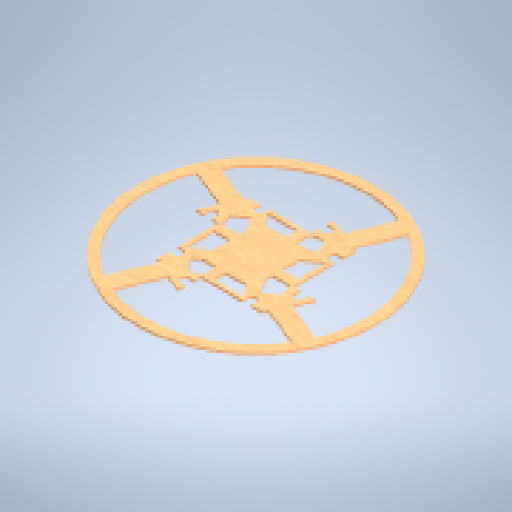
# Autodesk Inventor part: plate
Saved by Autodesk Inventor 2024.1 (Build 281209000, 209)
## iProperties
Created: 2024-07-03
Part Number: plate
Material: 木材 (サクラ材)
Document SubType Name: Modeling
Designer: hibik
Density: 0.63 g/cm^3
Appearance: サクラ材 - ナチュラル 抑えた光沢
Author: hibik
Autodesk Inventor part; units mm, degrees
ref_plane "YZ Plane" through (0, 0, 0) normal (1, 0, 0) x (0, 1, 0)
ref_plane "XZ Plane" through (0, 0, 0) normal (0, 1, 0) x (-1, 0, 0)
ref_plane "XY Plane" through (0, 0, 0) normal (0, 0, 1) x (1, 0, 0)
sketch "スケッチ1" plane through (0, 0, 0) normal (0, 1, 0) x (-1, 0, 0)
  line L0 (26.5, 31.5) -> (-26.5, 31.5)
  line L1 (-26.5, 31.5) -> (-26.5, -31.5)
  line L2 (-26.5, -31.5) -> (26.5, -31.5)
  line L3 (26.5, -31.5) -> (26.5, 31.5)
  line L4 (26.5, 31.5) -> (-26.5, -31.5) construction
  line L5 (-26.5, 31.5) -> (26.5, -31.5) construction
  point P0 (0, 0)
  dimension "d0" = 53
  dimension "d1" = 63
  constraints: 12 end point, 2 midpoint, 2 parallel, 1 horizontal, 1 perpendicular
  measures "d0" distance of L2.end L1.end
  measures "d1" distance of L1.end L0.end
extrude "押し出し1" add sketch "スケッチ1" along normal blind 2.5
sketch "スケッチ6" plane through (0, 0, 0) normal (0, -1, 0) x (1, 0, 0)
  arc A0 (26.3287, -65.2977) -> (29.0118, -58.5429) centre (24.4787, -60.6525) ccw projected
  line L0 (26.3287, -65.2977) -> (44.15, -58.2) projected
  line L1 (44.15, -54.8) -> (44.15, -58.2) projected
  line L2 (46.15, -54.8) -> (44.15, -54.8) projected
  line L3 (46.15, -54.8) -> (48, -54.8) projected
  line L4 (48, -43.3721) -> (48, -54.8) projected
  line L5 (48, -43.3721) -> (43, -43.3721) projected
  arc A1 (40.1241, -42.4623) -> (43, -43.3721) centre (43, -38.3721) ccw projected
  line L6 (40.1241, -42.4623) -> (42.3111, -44) projected
  arc A2 (36.5717, -56.5915) -> (42.3111, -44) centre (32.8717, -47.3012) ccw projected
  line L7 (36.5717, -56.5915) -> (32.1435, -58.3551) projected
  arc A3 (29.0118, -58.5429) -> (32.1435, -58.3551) centre (30.2935, -53.7099) ccw projected
  line L8 (-26.5, 18.6328) -> (-26.5, 0) projected
  line L9 (-26.5, 0) -> (-44, 0) projected
  line L10 (-44, 0) -> (-44, 30.9375) projected
  line L11 (-44, 30.9375) -> (-26.5, 18.6328) projected
  line L12 (22.5, 27.5) -> (22.5, -27.5) projected
  line L13 (22.5, -27.5) -> (-22.5, -27.5) projected
  line L14 (-22.5, -27.5) -> (-22.5, 27.5) projected
  line L15 (-22.5, 27.5) -> (22.5, 27.5) projected
  line L16 (22.1484, 31.5) -> (0, 31.5) projected
  line L17 (0, 31.5) -> (0, 44) projected
  line L18 (0, 44) -> (30.9375, 44) projected
  line L19 (30.9375, 44) -> (22.1484, 31.5) projected
  line L20 (26.5, -18.6328) -> (26.5, 0) projected
  line L21 (26.5, 0) -> (44, 0) projected
  line L22 (44, 0) -> (44, -30.9375) projected
  line L23 (44, -30.9375) -> (26.5, -18.6328) projected
  line L24 (-22.1484, -31.5) -> (0, -31.5) projected
  line L25 (0, -31.5) -> (0, -44) projected
  line L26 (0, -44) -> (-30.9375, -44) projected
  line L27 (-30.9375, -44) -> (-22.1484, -31.5) projected
  arc A4 (25.7604, -55.8196) -> (19.4893, -60.3263) centre (24.4787, -60.6525) ccw projected
  arc A5 (25.6484, -55.56) -> (25.7604, -55.8196) centre (30.2935, -53.7099) ccw projected
  arc A6 (25.6484, -55.56) -> (14.5, -48) centre (14.5, -60) ccw projected
  arc A7 (9.5, -43) -> (14.5, -48) centre (14.5, -43) ccw projected
  line L28 (9.5, -43) -> (9.5, -31.5) projected
  line L29 (9.5, -31.5) -> (24.5333, -31.5) projected
  line L30 (24.5333, -31.5) -> (40.1241, -42.4623) projected
  arc A8 (39.1622, -35.1673) -> (40.1241, -42.4623) centre (43, -38.3721) ccw projected
  circle A9 centre (35.3243, -31.9624) radius 5 projected
  arc A10 (43, -33.3721) -> (39.1622, -35.1673) centre (43, -38.3721) ccw projected
  line L31 (43, -33.3721) -> (48, -33.3721) projected
  line L32 (48, -19.5) -> (48, -33.3721) projected
  line L33 (50, -19.5) -> (48, -19.5) projected
  line L34 (50, -19.5) -> (50, 4.5) projected
  line L35 (48, 4.5) -> (50, 4.5) projected
  line L36 (48, 9.5) -> (48, 4.5) projected
  line L37 (53, 9.5) -> (48, 9.5) projected
  line L38 (53, 7.5) -> (53, 9.5) projected
  line L39 (53, 7.5) -> (67, 7.5) projected
  line L40 (67, 9.5) -> (67, 7.5) projected
  line L41 (72, 9.5) -> (67, 9.5) projected
  line L42 (72, 9.5) -> (65.2977, 26.3287) projected
  arc A11 (60.3263, 19.4893) -> (65.2977, 26.3287) centre (60.6525, 24.4787) ccw projected
  circle A12 centre (60, 14.5) radius 5 projected
  arc A13 (55.8196, 25.7604) -> (60.3263, 19.4893) centre (60.6525, 24.4787) ccw projected
  arc A14 (55.56, 25.6484) -> (55.8196, 25.7604) centre (53.7099, 30.2935) ccw projected
  arc A15 (55.56, 25.6484) -> (48, 14.5) centre (60, 14.5) ccw projected
  arc A16 (43, 9.5) -> (48, 14.5) centre (43, 14.5) ccw projected
  line L43 (43, 9.5) -> (26.5, 9.5) projected
  line L44 (26.5, 9.5) -> (26.5, 17.4222) projected
  line L45 (26.5, 17.4222) -> (42.4623, 40.1241) projected
  arc A17 (35.1673, 39.1622) -> (42.4623, 40.1241) centre (38.3721, 43) ccw projected
  circle A18 centre (31.9624, 35.3243) radius 5 projected
  arc A19 (33.3721, 43) -> (35.1673, 39.1622) centre (38.3721, 43) ccw projected
  line L46 (33.3721, 43) -> (33.3721, 48) projected
  line L47 (19.5, 48) -> (33.3721, 48) projected
  line L48 (19.5, 50) -> (19.5, 48) projected
  line L49 (19.5, 50) -> (-4.5, 50) projected
  line L50 (-4.5, 48) -> (-4.5, 50) projected
  line L51 (-9.5, 48) -> (-4.5, 48) projected
  line L52 (-9.5, 53) -> (-9.5, 48) projected
  line L53 (-7.5, 53) -> (-9.5, 53) projected
  line L54 (-7.5, 53) -> (-7.5, 67) projected
  line L55 (-9.5, 67) -> (-7.5, 67) projected
  line L56 (-9.5, 72) -> (-9.5, 67) projected
  line L57 (-9.5, 72) -> (-26.3287, 65.2977) projected
  arc A20 (-19.4893, 60.3263) -> (-26.3287, 65.2977) centre (-24.4787, 60.6525) ccw projected
  circle A21 centre (-14.5, 60) radius 5 projected
  arc A22 (-25.7604, 55.8196) -> (-19.4893, 60.3263) centre (-24.4787, 60.6525) ccw projected
  arc A23 (-25.6484, 55.56) -> (-25.7604, 55.8196) centre (-30.2935, 53.7099) ccw projected
  arc A24 (-25.6484, 55.56) -> (-14.5, 48) centre (-14.5, 60) ccw projected
  arc A25 (-9.5, 43) -> (-14.5, 48) centre (-14.5, 43) ccw projected
  line L58 (-9.5, 43) -> (-9.5, 31.5) projected
  line L59 (-9.5, 31.5) -> (-24.5333, 31.5) projected
  line L60 (-24.5333, 31.5) -> (-40.1241, 42.4623) projected
  arc A26 (-39.1622, 35.1673) -> (-40.1241, 42.4623) centre (-43, 38.3721) ccw projected
  circle A27 centre (-35.3243, 31.9624) radius 5 projected
  arc A28 (-43, 33.3721) -> (-39.1622, 35.1673) centre (-43, 38.3721) ccw projected
  line L61 (-43, 33.3721) -> (-48, 33.3721) projected
  line L62 (-48, 19.5) -> (-48, 33.3721) projected
  line L63 (-50, 19.5) -> (-48, 19.5) projected
  line L64 (-50, 19.5) -> (-50, -4.5) projected
  line L65 (-48, -4.5) -> (-50, -4.5) projected
  line L66 (-48, -9.5) -> (-48, -4.5) projected
  line L67 (-53, -9.5) -> (-48, -9.5) projected
  line L68 (-53, -7.5) -> (-53, -9.5) projected
  line L69 (-53, -7.5) -> (-67, -7.5) projected
  line L70 (-67, -9.5) -> (-67, -7.5) projected
  line L71 (-72, -9.5) -> (-67, -9.5) projected
  line L72 (-72, -9.5) -> (-65.2977, -26.3287) projected
  arc A29 (-60.3263, -19.4893) -> (-65.2977, -26.3287) centre (-60.6525, -24.4787) ccw projected
  circle A30 centre (-60, -14.5) radius 5 projected
  arc A31 (-55.8196, -25.7604) -> (-60.3263, -19.4893) centre (-60.6525, -24.4787) ccw projected
  arc A32 (-55.56, -25.6484) -> (-55.8196, -25.7604) centre (-53.7099, -30.2935) ccw projected
  arc A33 (-55.56, -25.6484) -> (-48, -14.5) centre (-60, -14.5) ccw projected
  arc A34 (-43, -9.5) -> (-48, -14.5) centre (-43, -14.5) ccw projected
  line L73 (-43, -9.5) -> (-26.5, -9.5) projected
  line L74 (-26.5, -9.5) -> (-26.5, -17.4222) projected
  line L75 (-26.5, -17.4222) -> (-42.4623, -40.1241) projected
  arc A35 (-35.1673, -39.1622) -> (-42.4623, -40.1241) centre (-38.3721, -43) ccw projected
  circle A36 centre (-31.9624, -35.3243) radius 5 projected
  arc A37 (-33.3721, -43) -> (-35.1673, -39.1622) centre (-38.3721, -43) ccw projected
  line L76 (-33.3721, -43) -> (-33.3721, -48) projected
  line L77 (-19.5, -48) -> (-33.3721, -48) projected
  line L78 (-19.5, -50) -> (-19.5, -48) projected
  line L79 (-19.5, -50) -> (4.5, -50) projected
  line L80 (4.5, -48) -> (4.5, -50) projected
  line L81 (9.5, -48) -> (4.5, -48) projected
  line L82 (9.5, -53) -> (9.5, -48) projected
  line L83 (7.5, -53) -> (9.5, -53) projected
  line L84 (7.5, -53) -> (7.5, -67) projected
  line L85 (9.5, -67) -> (7.5, -67) projected
  line L86 (9.5, -72) -> (9.5, -67) projected
  line L87 (9.5, -72) -> (26.3287, -65.2977) projected
  arc A38 (19.4893, -60.3263) -> (26.3287, -65.2977) centre (24.4787, -60.6525) ccw projected
  circle A39 centre (14.5, -60) radius 5 projected
  arc A40 (-65.2977, -26.3287) -> (-58.5429, -29.0118) centre (-60.6525, -24.4787) ccw projected
  line L88 (-65.2977, -26.3287) -> (-58.2, -44.15) projected
  line L89 (-54.8, -44.15) -> (-58.2, -44.15) projected
  line L90 (-54.8, -46.15) -> (-54.8, -44.15) projected
  line L91 (-54.8, -46.15) -> (-54.8, -48) projected
  line L92 (-43.3721, -48) -> (-54.8, -48) projected
  line L93 (-43.3721, -48) -> (-43.3721, -43) projected
  arc A41 (-42.4623, -40.1241) -> (-43.3721, -43) centre (-38.3721, -43) ccw projected
  line L94 (-42.4623, -40.1241) -> (-44, -42.3111) projected
  arc A42 (-56.5915, -36.5717) -> (-44, -42.3111) centre (-47.3012, -32.8717) ccw projected
  line L95 (-56.5915, -36.5717) -> (-58.3551, -32.1435) projected
  arc A43 (-58.5429, -29.0118) -> (-58.3551, -32.1435) centre (-53.7099, -30.2935) ccw projected
  arc A44 (-26.3287, 65.2977) -> (-29.0118, 58.5429) centre (-24.4787, 60.6525) ccw projected
  line L96 (-26.3287, 65.2977) -> (-44.15, 58.2) projected
  line L97 (-44.15, 54.8) -> (-44.15, 58.2) projected
  line L98 (-46.15, 54.8) -> (-44.15, 54.8) projected
  line L99 (-46.15, 54.8) -> (-48, 54.8) projected
  line L100 (-48, 43.3721) -> (-48, 54.8) projected
  line L101 (-48, 43.3721) -> (-43, 43.3721) projected
  arc A45 (-40.1241, 42.4623) -> (-43, 43.3721) centre (-43, 38.3721) ccw projected
  line L102 (-40.1241, 42.4623) -> (-42.3111, 44) projected
  arc A46 (-36.5717, 56.5915) -> (-42.3111, 44) centre (-32.8717, 47.3012) ccw projected
  line L103 (-36.5717, 56.5915) -> (-32.1435, 58.3551) projected
  arc A47 (-29.0118, 58.5429) -> (-32.1435, 58.3551) centre (-30.2935, 53.7099) ccw projected
  arc A48 (65.2977, 26.3287) -> (58.5429, 29.0118) centre (60.6525, 24.4787) ccw projected
  line L104 (65.2977, 26.3287) -> (58.2, 44.15) projected
  line L105 (54.8, 44.15) -> (58.2, 44.15) projected
  line L106 (54.8, 46.15) -> (54.8, 44.15) projected
  line L107 (54.8, 46.15) -> (54.8, 48) projected
  line L108 (43.3721, 48) -> (54.8, 48) projected
  line L109 (43.3721, 48) -> (43.3721, 43) projected
  arc A49 (42.4623, 40.1241) -> (43.3721, 43) centre (38.3721, 43) ccw projected
  line L110 (42.4623, 40.1241) -> (44, 42.3111) projected
  arc A50 (56.5915, 36.5717) -> (44, 42.3111) centre (47.3012, 32.8717) ccw projected
  line L111 (56.5915, 36.5717) -> (58.3551, 32.1435) projected
  arc A51 (58.5429, 29.0118) -> (58.3551, 32.1435) centre (53.7099, 30.2935) ccw projected
  line L112 (35.3243, -31.9624) -> (14.5, -60)
  line L113 (-31.9624, -35.3243) -> (-60, -14.5)
  line L114 (-35.3243, 31.9624) -> (-14.5, 60)
  line L115 (60, 14.5) -> (31.9624, 35.3243)
  line L116 (-48, -9.5) -> (-48, 33.3721) projected
  line L117 (9.5, -48) -> (-33.3721, -48) projected
  line L118 (48, 9.5) -> (48, -33.3721) projected
  line L119 (-9.5, 48) -> (33.3721, 48) projected
  circle A52 centre (-60, -14.5) radius 1.55 projected
  circle A53 centre (-43, 38.3721) radius 1.55 projected
  circle A54 centre (-71.5, 53.2) radius 1.55 projected
  line L120 (-51.7493, 27.3) -> (-63.2507, 27.3) projected
  line L121 (-63.2507, 27.3) -> (-57.5, 36.8845) projected
  line L122 (-57.5, 36.8845) -> (-51.7493, 27.3) projected
  line L123 (-50, -4.5) -> (-57.5556, 7.5) projected
  line L124 (-57.5556, 7.5) -> (-50, 19.5) projected
  line L125 (-50, 19.5) -> (-50, -4.5) projected
  line L126 (-70, 19.5) -> (-62.4444, 7.5) projected
  line L127 (-62.4444, 7.5) -> (-70, -4.5) projected
  line L128 (-70, -4.5) -> (-70, 19.5) projected
  line L129 (-50, 49.3845) -> (-50, 30.2155) projected
  line L130 (-50, 30.2155) -> (-55.7507, 39.8) projected
  line L131 (-55.7507, 39.8) -> (-50, 49.3845) projected
  line L132 (-59.2493, 39.8) -> (-65, 30.2155) projected
  line L133 (-65, 30.2155) -> (-65, 49.3845) projected
  line L134 (-65, 49.3845) -> (-59.2493, 39.8) projected
  line L135 (-53, 22.5) -> (-60, 11.3824) projected
  line L136 (-60, 11.3824) -> (-67, 22.5) projected
  line L137 (-67, 22.5) -> (-53, 22.5) projected
  line L138 (-67, -7.5) -> (-60, 3.6176) projected
  line L139 (-60, 3.6176) -> (-53, -7.5) projected
  line L140 (-53, -7.5) -> (-67, -7.5) projected
  line L141 (-51.7493, 52.3) -> (-57.5, 42.7155) projected
  line L142 (-57.5, 42.7155) -> (-63.2507, 52.3) projected
  line L143 (-63.2507, 52.3) -> (-51.7493, 52.3) projected
  line L144 (-66.5, 58.3) -> (-66.5, 58.2) projected
  line L145 (-66.5, 58.2) -> (-71.5, 58.2) projected
  arc A55 (-71.5, 58.2) -> (-71.5, 48.2) centre (-71.5, 53.2) ccw projected
  line L146 (-71.5, 48.2) -> (-66.5, 48.2) projected
  line L147 (-66.5, 48.2) -> (-66.5, 27.3) projected
  line L148 (-66.5, 27.3) -> (-72, 27.3) projected
  line L149 (-72, 27.3) -> (-72, -9.5) projected
  line L150 (-72, -9.5) -> (-65, -9.5) projected
  line L151 (-65, -9.5) -> (-65, -14.5) projected
  arc A56 (-65, -14.5) -> (-55, -14.5) centre (-60, -14.5) ccw projected
  line L152 (-55, -14.5) -> (-55, -9.5) projected
  line L153 (-55, -9.5) -> (-48, -9.5) projected
  line L154 (-48, -9.5) -> (-48, 33.3721) projected
  line L155 (-48, 33.3721) -> (-43, 33.3721) projected
  arc A57 (-43, 33.3721) -> (-43, 43.3721) centre (-43, 38.3721) ccw projected
  line L156 (-43, 43.3721) -> (-48, 43.3721) projected
  line L157 (-48, 43.3721) -> (-48, 54.8) projected
  line L158 (-48, 54.8) -> (-44.1513, 54.8) projected
  line L159 (-44.1513, 58.3) -> (-44.1513, 54.8) projected
  line L160 (-66.5, 58.3) -> (-44.1513, 58.3) projected
  circle A58 centre (14.5, -60) radius 1.55 projected
  circle A59 centre (-38.3721, -43) radius 1.55 projected
  circle A60 centre (-53.2, -71.5) radius 1.55 projected
  line L161 (-27.3, -51.7493) -> (-27.3, -63.2507) projected
  line L162 (-27.3, -63.2507) -> (-36.8845, -57.5) projected
  line L163 (-36.8845, -57.5) -> (-27.3, -51.7493) projected
  line L164 (4.5, -50) -> (-7.5, -57.5556) projected
  line L165 (-7.5, -57.5556) -> (-19.5, -50) projected
  line L166 (-19.5, -50) -> (4.5, -50) projected
  line L167 (-19.5, -70) -> (-7.5, -62.4444) projected
  line L168 (-7.5, -62.4444) -> (4.5, -70) projected
  line L169 (4.5, -70) -> (-19.5, -70) projected
  line L170 (-49.3845, -50) -> (-30.2155, -50) projected
  line L171 (-30.2155, -50) -> (-39.8, -55.7507) projected
  line L172 (-39.8, -55.7507) -> (-49.3845, -50) projected
  line L173 (-39.8, -59.2493) -> (-30.2155, -65) projected
  line L174 (-30.2155, -65) -> (-49.3845, -65) projected
  line L175 (-49.3845, -65) -> (-39.8, -59.2493) projected
  line L176 (-22.5, -53) -> (-11.3824, -60) projected
  line L177 (-11.3824, -60) -> (-22.5, -67) projected
  line L178 (-22.5, -67) -> (-22.5, -53) projected
  line L179 (7.5, -67) -> (-3.6176, -60) projected
  line L180 (-3.6176, -60) -> (7.5, -53) projected
  line L181 (7.5, -53) -> (7.5, -67) projected
  line L182 (-52.3, -51.7493) -> (-42.7155, -57.5) projected
  line L183 (-42.7155, -57.5) -> (-52.3, -63.2507) projected
  line L184 (-52.3, -63.2507) -> (-52.3, -51.7493) projected
  line L185 (-58.3, -66.5) -> (-58.2, -66.5) projected
  line L186 (-58.2, -66.5) -> (-58.2, -71.5) projected
  arc A61 (-58.2, -71.5) -> (-48.2, -71.5) centre (-53.2, -71.5) ccw projected
  line L187 (-48.2, -71.5) -> (-48.2, -66.5) projected
  line L188 (-48.2, -66.5) -> (-27.3, -66.5) projected
  line L189 (-27.3, -66.5) -> (-27.3, -72) projected
  line L190 (-27.3, -72) -> (9.5, -72) projected
  line L191 (9.5, -72) -> (9.5, -65) projected
  line L192 (9.5, -65) -> (14.5, -65) projected
  arc A62 (14.5, -65) -> (14.5, -55) centre (14.5, -60) ccw projected
  line L193 (14.5, -55) -> (9.5, -55) projected
  line L194 (9.5, -55) -> (9.5, -48) projected
  line L195 (9.5, -48) -> (-33.3721, -48) projected
  line L196 (-33.3721, -48) -> (-33.3721, -43) projected
  arc A63 (-33.3721, -43) -> (-43.3721, -43) centre (-38.3721, -43) ccw projected
  line L197 (-43.3721, -43) -> (-43.3721, -48) projected
  line L198 (-43.3721, -48) -> (-54.8, -48) projected
  line L199 (-54.8, -48) -> (-54.8, -44.1513) projected
  line L200 (-58.3, -44.1513) -> (-54.8, -44.1513) projected
  line L201 (-58.3, -66.5) -> (-58.3, -44.1513) projected
  circle A64 centre (60, 14.5) radius 1.55 projected
  circle A65 centre (43, -38.3721) radius 1.55 projected
  circle A66 centre (71.5, -53.2) radius 1.55 projected
  line L202 (51.7493, -27.3) -> (63.2507, -27.3) projected
  line L203 (63.2507, -27.3) -> (57.5, -36.8845) projected
  line L204 (57.5, -36.8845) -> (51.7493, -27.3) projected
  line L205 (50, 4.5) -> (57.5556, -7.5) projected
  line L206 (57.5556, -7.5) -> (50, -19.5) projected
  line L207 (50, -19.5) -> (50, 4.5) projected
  line L208 (70, -19.5) -> (62.4444, -7.5) projected
  line L209 (62.4444, -7.5) -> (70, 4.5) projected
  line L210 (70, 4.5) -> (70, -19.5) projected
  line L211 (50, -49.3845) -> (50, -30.2155) projected
  line L212 (50, -30.2155) -> (55.7507, -39.8) projected
  line L213 (55.7507, -39.8) -> (50, -49.3845) projected
  line L214 (59.2493, -39.8) -> (65, -30.2155) projected
  line L215 (65, -30.2155) -> (65, -49.3845) projected
  line L216 (65, -49.3845) -> (59.2493, -39.8) projected
  line L217 (53, -22.5) -> (60, -11.3824) projected
  line L218 (60, -11.3824) -> (67, -22.5) projected
  line L219 (67, -22.5) -> (53, -22.5) projected
  line L220 (67, 7.5) -> (60, -3.6176) projected
  line L221 (60, -3.6176) -> (53, 7.5) projected
  line L222 (53, 7.5) -> (67, 7.5) projected
  line L223 (51.7493, -52.3) -> (57.5, -42.7155) projected
  line L224 (57.5, -42.7155) -> (63.2507, -52.3) projected
  line L225 (63.2507, -52.3) -> (51.7493, -52.3) projected
  line L226 (66.5, -58.3) -> (66.5, -58.2) projected
  line L227 (66.5, -58.2) -> (71.5, -58.2) projected
  arc A67 (71.5, -58.2) -> (71.5, -48.2) centre (71.5, -53.2) ccw projected
  line L228 (71.5, -48.2) -> (66.5, -48.2) projected
  line L229 (66.5, -48.2) -> (66.5, -27.3) projected
  line L230 (66.5, -27.3) -> (72, -27.3) projected
  line L231 (72, -27.3) -> (72, 9.5) projected
  line L232 (72, 9.5) -> (65, 9.5) projected
  line L233 (65, 9.5) -> (65, 14.5) projected
  arc A68 (65, 14.5) -> (55, 14.5) centre (60, 14.5) ccw projected
  line L234 (55, 14.5) -> (55, 9.5) projected
  line L235 (55, 9.5) -> (48, 9.5) projected
  line L236 (48, 9.5) -> (48, -33.3721) projected
  line L237 (48, -33.3721) -> (43, -33.3721) projected
  arc A69 (43, -33.3721) -> (43, -43.3721) centre (43, -38.3721) ccw projected
  line L238 (43, -43.3721) -> (48, -43.3721) projected
  line L239 (48, -43.3721) -> (48, -54.8) projected
  line L240 (48, -54.8) -> (44.1513, -54.8) projected
  line L241 (44.1513, -58.3) -> (44.1513, -54.8) projected
  line L242 (66.5, -58.3) -> (44.1513, -58.3) projected
  circle A70 centre (-14.5, 60) radius 1.55 projected
  circle A71 centre (38.3721, 43) radius 1.55 projected
  circle A72 centre (53.2, 71.5) radius 1.55 projected
  line L243 (27.3, 51.7493) -> (27.3, 63.2507) projected
  line L244 (27.3, 63.2507) -> (36.8845, 57.5) projected
  line L245 (36.8845, 57.5) -> (27.3, 51.7493) projected
  line L246 (-4.5, 50) -> (7.5, 57.5556) projected
  line L247 (7.5, 57.5556) -> (19.5, 50) projected
  line L248 (19.5, 50) -> (-4.5, 50) projected
  line L249 (19.5, 70) -> (7.5, 62.4444) projected
  line L250 (7.5, 62.4444) -> (-4.5, 70) projected
  line L251 (-4.5, 70) -> (19.5, 70) projected
  line L252 (49.3845, 50) -> (30.2155, 50) projected
  line L253 (30.2155, 50) -> (39.8, 55.7507) projected
  line L254 (39.8, 55.7507) -> (49.3845, 50) projected
  line L255 (39.8, 59.2493) -> (30.2155, 65) projected
  line L256 (30.2155, 65) -> (49.3845, 65) projected
  line L257 (49.3845, 65) -> (39.8, 59.2493) projected
  line L258 (22.5, 53) -> (11.3824, 60) projected
  line L259 (11.3824, 60) -> (22.5, 67) projected
  line L260 (22.5, 67) -> (22.5, 53) projected
  line L261 (-7.5, 67) -> (3.6176, 60) projected
  line L262 (3.6176, 60) -> (-7.5, 53) projected
  line L263 (-7.5, 53) -> (-7.5, 67) projected
  line L264 (52.3, 51.7493) -> (42.7155, 57.5) projected
  line L265 (42.7155, 57.5) -> (52.3, 63.2507) projected
  line L266 (52.3, 63.2507) -> (52.3, 51.7493) projected
  line L267 (58.3, 66.5) -> (58.2, 66.5) projected
  line L268 (58.2, 66.5) -> (58.2, 71.5) projected
  arc A73 (58.2, 71.5) -> (48.2, 71.5) centre (53.2, 71.5) ccw projected
  line L269 (48.2, 71.5) -> (48.2, 66.5) projected
  line L270 (48.2, 66.5) -> (27.3, 66.5) projected
  line L271 (27.3, 66.5) -> (27.3, 72) projected
  line L272 (27.3, 72) -> (-9.5, 72) projected
  line L273 (-9.5, 72) -> (-9.5, 65) projected
  line L274 (-9.5, 65) -> (-14.5, 65) projected
  arc A74 (-14.5, 65) -> (-14.5, 55) centre (-14.5, 60) ccw projected
  line L275 (-14.5, 55) -> (-9.5, 55) projected
  line L276 (-9.5, 55) -> (-9.5, 48) projected
  line L277 (-9.5, 48) -> (33.3721, 48) projected
  line L278 (33.3721, 48) -> (33.3721, 43) projected
  arc A75 (33.3721, 43) -> (43.3721, 43) centre (38.3721, 43) ccw projected
  line L279 (43.3721, 43) -> (43.3721, 48) projected
  line L280 (43.3721, 48) -> (54.8, 48) projected
  line L281 (54.8, 48) -> (54.8, 44.1513) projected
  line L282 (58.3, 44.1513) -> (54.8, 44.1513) projected
  line L283 (58.3, 66.5) -> (58.3, 44.1513) projected
  point P0 (0, 0)
  point P1 (31.8479, -36.6431)
  point P2 (21.6551, -50.3665)
  point P3 (36.6431, 31.8479)
  point P4 (50.3665, 21.6551)
  point P5 (-31.8479, 36.6431)
  point P6 (-21.6551, 50.3665)
  point P7 (-36.6431, -31.8479)
  point P8 (-50.3665, -21.6551)
  constraints: 8 end point, 4 other
extrude "押し出し6" add sketch "スケッチ6" against normal blind 2.5 contours A38 A4 A5 A6 L112 L30 L6 A2 L7 A3 A0 | A0 A3 L7 A2 L6 A1 L5 L4 L3 L2 L1 L0 | L87 L86 L191 L192 A39 A38 | A39 L112 A6 A5 A4 | L193 L194 L82 L81 L117 L77 L76 A37 A36 L113 L75 L74 L73 A34 A33 A30 L152 L153 L67 L66 L116 L62 L61 A28 A27 L114 L60 L59 L58 A25 A24 A21 L275 L276 L52 L51 L119 L47 L46 A19 A18 L115 L45 L44 L43 A16 A15 A12 L234 L235 L37 L36 L118 L32 L31 A10 A9 L112 L30 L29 L28 A7 A6 A39 | L30 L112 A9 A8 | A9 | L41 L232 L233 A12 A11 L42 | L88 A40 A43 L95 A42 L94 A41 L93 L92 L91 L90 L89 | A11 A13 A14 A15 L115 L45 L110 A50 L111 A51 A48 | A48 A51 L111 A50 L110 A49 L109 L108 L107 L106 L105 L104 | A36 | A35 L75 L113 A36 | L72 L71 L150 L151 A30 A29 | A29 A31 A32 A33 L113 L75 L94 A42 L95 A43 A40 | A12 L115 A15 A14 A13 | A30 L113 A33 A32 A31 | L115 A18 A17 L45 | A18 | L56 L273 L274 A21 A20 L57 | L96 A44 A47 L103 A46 L102 A45 L101 L100 L99 L98 L97 | A20 A22 A23 A24 L114 L60 L102 A46 L103 A47 A44 | A27 | A26 L60 L114 A27 | A21 L114 A24 A23 A22
sketch "スケッチ7" plane through (0, 0, 0) normal (0, -1, 0) x (1, 0, 0)
  circle A0 centre (0, 0) radius 115
  circle A1 centre (0, 0) radius 125
  line L0 (58.2, 44.15) -> (72, 9.5) projected
  line L1 (58.2, 44.15) -> (64.8601, 27.4275)
  line L2 (64.8601, 27.4275) -> (106.29, 43.9277)
  line L3 (106.29, 43.9277) -> (99.6299, 60.6502) construction
  line L4 (99.6299, 60.6502) -> (58.2, 44.15)
  line L5 (-27.4275, 64.8601) -> (-43.9277, 106.29)
  line L6 (-60.6502, 99.6299) -> (-44.15, 58.2)
  line L7 (-64.8601, -27.4275) -> (-106.29, -43.9277)
  line L8 (-99.6299, -60.6502) -> (-58.2, -44.15)
  line L9 (27.4275, -64.8601) -> (43.9277, -106.29)
  line L10 (60.6502, -99.6299) -> (44.15, -58.2)
  line L11 (-44.15, 58.2) -> (-27.4275, 64.8601)
  line L12 (-58.2, -44.15) -> (-64.8601, -27.4275)
  line L13 (44.15, -58.2) -> (27.4275, -64.8601)
  point P0 (106.2811, 43.9241)
  point P1 (60.0352, -98.0856)
  point P2 (43.9241, -106.2811)
  point P3 (-98.0856, -60.0352)
  point P4 (-106.2811, -43.9241)
  point P5 (-60.0352, 98.0856)
  point P6 (-43.9241, 106.2811)
  point P7 (98.0856, 60.0352)
  dimension "d22" = 230
  dimension "d23" = 250
  dimension "d24" = 18
  dimension "d27" = 360
  dimension "d31" = 360
  constraints: 26 end point, 2 centre point, 2 coincident, 2 parallel, 1 perpendicular, 1 point on line, 1 tangent, 38 other
  measures "d22" diameter of A0
  measures "d23" diameter of A1
  measures "d24" distance between parallel lines of L2 L4
extrude "押し出し7" add sketch "スケッチ7" against normal blind 2.5 contours L2 L0 L4 A0 | A0 L9 L13 L10 | L5 L11 L6 A0 | A0 L7 L12 L8 | A1
